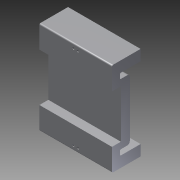
# Autodesk Inventor part: KR45H-A-Slider Spacer
Saved by Autodesk Inventor 2011 SP1 (Build 150282100, 282)
## iProperties
Created: 2013-10-24
Part Number: KR45H-A-Slider Spacer
Catalog Web Link: www.cadenas.de
Description: LM Guide Actuator - Slider Spacer-KR
Vendor: THK
Document SubType Name: Modeling
Designer: PARTuser1
Manufacturer: THK
Density: 1 g/cm^3
Category: PARTsolutions
Company: THK
Title: KR45H-A-Slider Spacer
Author: Cadenas PARTsolutions
Comments: KR
PSOL_IDENT_0: {$CADENAS_DATA\23d-libs\thk\lm_guide_actuator\type_kr\parts\lm_g_a_kr_slider_spacer.prj},216 {VTYP=3
PSOL_IDENT_1: D},{NB=KR45H-A-Slider Spacer},{LINA=KR45H-A-Slider Spacer},{NN=LM Guide Actuator - Slider Spacer},{D
PSOL_IDENT_2: ATE=17.05.2010 06:34:46},{GEOMDATE=07.11.2007 11:59:00},{VERSION=},{LINEID=60},{LINESUBID=-1},{WBVAR
PSOL_IDENT_3: =TYPE1}  {NB=KR45H-A-Slider Spacer},{LINA=KR45H-A-Slider Spacer},{KT=DUMMY},{ORDER=KR45H},{XTYPE2=6.
PSOL_IDENT_4: 000},{TYPE1=A},{TYPE2='A','B','C','D'},{XTYPE=1}
CNS_NT: KR
CNS_NB: KR45H-A-Slider Spacer
CNS_NBSYN: $ORDER.-$TYPE1.-Slider Spacer
CNS_LINA: KR45H-A-Slider Spacer
CNS_ORDER: KR45H
CNS_XTYPE2: 6.000
CNS_TYPE1: A
CNS_TYPE2: 'A','B','C','D'
CNS_XTYPE: 1.000
SUPPLIER: THK
ARTICLENO: KR45H-A-Slider Spacer
BOMINFO: KR45H-A-Slider Spacer
CREATOR: CADENAS GmbH
Autodesk Inventor part; units mm, degrees
sketch "Sketch_1" plane through (0, 0, 0) normal (1, 0, 0) x (0, 1, 0)
  line L0 (22, 52) -> (-8.5, 52)
  arc A0 (-8.5, 52) -> (-10, 50.5) centre (-8.5, 50.5) ccw
  line L1 (-10, 50.5) -> (-10, 26.75)
  line L2 (-10, 26.75) -> (0, 26.75)
  line L3 (0, 26.75) -> (0, -26.75)
  line L4 (0, -26.75) -> (-10, -26.75)
  line L5 (-10, -26.75) -> (-10, -50.5)
  arc A1 (-10, -50.5) -> (-8.5, -52) centre (-8.5, -50.5) ccw
  line L6 (-8.5, -52) -> (22, -52)
  line L7 (22, -52) -> (22, -40)
  line L8 (22, -40) -> (0, -40)
  arc A2 (-1, -39) -> (0, -40) centre (0, -39) ccw
  line L9 (-1, -39) -> (-1, -35)
  arc A3 (0, -34) -> (-1, -35) centre (0, -35) ccw
  line L10 (0, -34) -> (7, -34)
  arc A4 (7, -34) -> (10, -31) centre (7, -31) ccw
  line L11 (10, -31) -> (10, 31)
  arc A5 (10, 31) -> (7, 34) centre (7, 31) ccw
  line L12 (7, 34) -> (0, 34)
  arc A6 (-1, 35) -> (0, 34) centre (0, 35) ccw
  line L13 (-1, 35) -> (-1, 39)
  arc A7 (0, 40) -> (-1, 39) centre (0, 39) ccw
  line L14 (0, 40) -> (22, 40)
  line L15 (22, 40) -> (22, 52)
  constraints: 32 end point, 16 point on circle, 8 centre point
extrude "Extrusion1" add sketch "Sketch_1" along normal mid plane 81
sketch "Sketch2" plane through (-40.5, 22, 40) normal (0, 1, 0) x (1, 0, 0)
  point P0 (17.5, -6)
hole "Drilling 1" at (-23, 22, 46) direction (0, -1, 0) diameter 4.917 depth 13.5 tip angle 140 countersink diameter 6 countersink angle 90 thread size "M6x1" class "6H" standard "ISO Metric profile"
pattern_linear "Rectangular Pattern1" count 2 spacing 46 along (1, 0, 0) count 2 spacing 92 along (0, 0, -1) of "Drilling 1"
sketch "Sketch3" plane through (-40.5, -10, 50.5) normal (0, -1, 0) x (1, 0, 0)
  point P0 (38, -3.5)
hole "Drilling 2" at (-2.5, -10, 47) direction (0, 1, 0) diameter 2.1129 depth 6 tip angle 140 countersink diameter 2.6 countersink angle 90 thread size "M2.6x0.45" class "6H" standard "ISO Metric profile"
pattern_linear "Rectangular Pattern2" count 2 spacing 5 along (1, 0, 0) count 2 spacing 94 along (0, 0, -1) of "Drilling 2"
ref_plane "slider_spacer_sensor_dog_XY" through (0, -10, 47) normal (0, 1, 0) x (1, 0, 0)
ref_plane "slider_spacer_sensor_dog_YZ" through (0, -10, 47) normal (1, 0, 0) x (0, 0, -1)
ref_plane "slider_spacer_sensor_dog_ZX" through (0, -10, 47) normal (0, 0, -1) x (0, 1, 0)
ref_plane "slider_spacer_slider_XY" through (0, 0, 0) normal (0, 1, 0) x (1, 0, 0)
ref_plane "slider_spacer_slider_YZ" through (0, 0, 0) normal (1, 0, 0) x (0, 0, -1)
ref_plane "slider_spacer_slider_ZX" through (0, 0, 0) normal (0, 0, -1) x (0, 1, 0)
body "Solid1"
